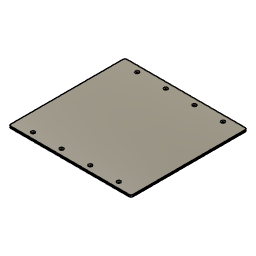
deck_panel_front_m3_countersunk_screws (Autodesk Fusion 360 design; units mm, degrees)
Autodesk Fusion 360 part; units mm, degrees
sketch "Sketch1" plane through (0, 0, 0) normal (0, 0, 1) x (1, 0, 0)
  line L0 (0, 0) -> (200, 0)
  line L1 (200, 0) -> (200, 190)
  line L2 (200, 190) -> (0, 190)
  line L3 (0, 190) -> (0, 0)
  dimension "d1" = 200
  dimension "d2" = 190
  constraint horizontal L0
  constraint vertical L1
  constraint horizontal L2
  constraint vertical L3
  constraint coincident L0.start L3.end
  measures "d1" distance of L1.end L2.end
  measures "d2" distance of L0.start L2.end
extrude "Extrude1" add sketch "Sketch1" along normal blind 3
sketch "Sketch2" plane through (0, 0, 3) normal (0, 0, 1) x (-1, 0, 0)
  line L0 (0, -190) -> (0, 0)
  line L1 (0, 0) -> (-200, 0)
  line L2 (-200, 0) -> (-200, -190)
  line L3 (-200, -190) -> (0, -190)
  point P0 (-30.003, -10.01)
  point P1 (-76.67, -10.01)
  point P2 (-123.337, -10.01)
  point P3 (-170.004, -10.01)
  point P4 (-30.003, -180.01)
  point P5 (-76.67, -180.01)
  point P6 (-123.337, -180.01)
  point P7 (-170.004, -180.01)
  dimension "d5" = 30.003
  dimension "d6" = 10.01
  dimension "d9" = 46.667
  dimension "d10" = 170
  measures "d5" distance of L0 P0
  measures "d6" distance of L1 P0
hole "Hole1" at (30.003, 10.01, 3) at (76.67, 10.01, 3) at (123.337, 10.01, 3) at (170.004, 10.01, 3) at (170.004, 180.01, 3) at (123.337, 180.01, 3) at (76.67, 180.01, 3) at (30.003, 180.01, 3) direction (0, 0, -1) diameter 3.4 end through all countersink diameter 6 countersink angle 90
fillet "Fillet2" radius 4 4 edges at (0, 190, 1.5) (200, 190, 1.5) (200, 0, 1.5) (0, 0, 1.5)
chamfer "Chamfer1" distance 0.4 angle 45 4 edges at (100, 0, 3) (0, 95, 3) (100, 190, 3) (200, 95, 3) 1 faces at (139.0678, 122.8044, 0)
equation "d5 = 28.303 mm + 1.7 mm"
equation "d6 = 8.310 mm + 1.7 mm"
